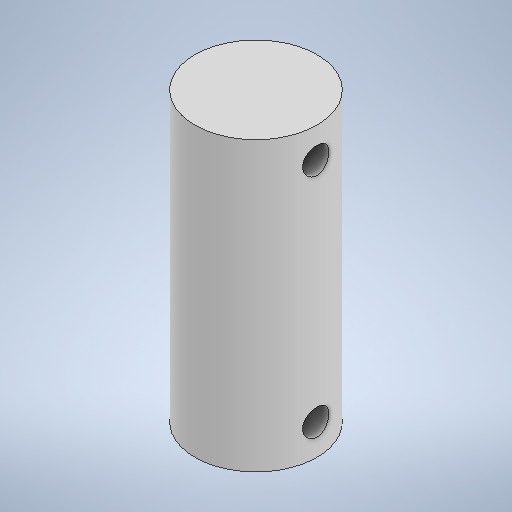
# Autodesk Inventor part: 2
Saved by Autodesk Inventor 2025 (Build 290162010, 162A)
## iProperties
Created: 2024-05-28
Part Number: 2
Material: Generic
Document SubType Name: Modeling
Designer: Fabri
Density: 1 g/cm^3
Appearance: Default
Author: Fabri
Autodesk Inventor part; units mm, degrees
ref_plane "XZ Plane" through (0, 0, 0) normal (0, 1, 0) x (-1, 0, 0)
ref_plane "XY Plane" through (0, 0, 0) normal (0, 0, 1) x (1, 0, 0)
sketch "Sketch1" plane through (0, 0, 0) normal (0, 1, 0) x (-1, 0, 0)
  circle A0 centre (0, 0) radius 7
  dimension "d0" = 14
  constraints: 1 centre point, 1 coincident
  measures "d0" diameter of A0
extrude "Extrusion1" add sketch "Sketch1" along normal blind 33
ref_plane "Work Plane1" through (7, 0, 0) normal (1, 0, 0) x (0, 1, 0)
sketch "Sketch2" plane through (7, 0, 0) normal (1, 0, 0) x (0, 1, 0)
  line L0 (33, -7) -> (33, 7) projected
  line L1 (0, -7) -> (0, 7) projected
  point P0 (0, 0)
  point P1 (29.5, 0)
  point P2 (3.5, 0)
  dimension "d4" = 3.5
  dimension "d5" = 3.5
  constraints: 2 horizontal alignment
  measures "d4" distance from line of L0 point (29.5, 0)
  measures "d5" distance from line of L1 point (3.5, 0)
hole "Hole1" at (7, 29.5, 0) at (7, 3.5, 0) direction (-1, 0, 0) diameter 3 end through all
equation "\"d5\" = d4"
body "Solid1"
